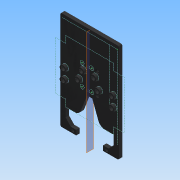
# Autodesk Inventor part: fix3
Saved by Autodesk Inventor 2015 (Build 190159000, 159)
## iProperties
Created: 2015-06-10
Part Number: fix3
Material: Générique
Document SubType Name: Modeling
Designer: Gregwar
Density: 1 g/cm^3
Appearance: Par défaut
Author: Gregwar
Autodesk Inventor part; units mm, degrees
ref_plane "YZ Plane" through (0, 0, 0) normal (1, 0, 0) x (0, 1, 0)
ref_plane "XZ Plane" through (0, 0, 0) normal (0, 1, 0) x (-1, 0, 0)
ref_plane "XY Plane" through (0, 0, 0) normal (0, 0, 1) x (1, 0, 0)
sketch "Esquisse1" plane through (0, 0, 0) normal (0, 1, 0) x (-1, 0, 0)
  line L0 (0, 0) -> (80, 0) construction
  line L1 (80, 0) -> (80, -120) construction
  line L2 (80, -120) -> (0, -120) construction
  line L3 (0, -120) -> (0, 0) construction
  line L4 (40, -120) -> (40, 0) construction
  line L5 (77.0201, -120) -> (40, -28.372) construction
  line L6 (75, 0) -> (75, -120) construction
  circle A0 centre (75, -60) radius 2.5 construction
  circle A1 centre (75, -75) radius 2.5 construction
  circle A2 centre (54.3966, -64.0049) radius 2.5 construction
  circle A3 centre (48.7775, -50.0971) radius 2.5 construction
  circle A4 centre (75, -20) radius 2 construction
  circle A5 centre (75, -5) radius 2 construction
  circle A6 centre (75, -115) radius 2 construction
  circle A7 centre (69.3809, -101.0922) radius 2 construction
  line L7 (75, -115) -> (69.3809, -101.0922) construction
  line L8 (52.7921, -43.0825) -> (41.0169, -47.84) construction
  line L9 (82.7607, -117.2572) -> (70.9854, -122.0147) construction
  line L10 (70.9854, -122.0147) -> (41.0169, -47.84) construction
  line L11 (82.7607, -117.2572) -> (52.7921, -43.0825) construction
  line L12 (54.3966, -64.0049) -> (69.3809, -101.0922) construction
  line L13 (67.7764, -80.1698) -> (56.0012, -84.9273) construction
  line L14 (81.35, 0) -> (68.65, 0) construction
  line L15 (68.65, 0) -> (68.65, -80) construction
  line L16 (68.65, -80) -> (81.35, -80) construction
  line L17 (81.35, -80) -> (81.35, 0) construction
  line L18 (75, 0) -> (75, -80) construction
  line L19 (75, -20) -> (75, -60) construction
  line L20 (2.9799, -120) -> (40, -28.372) construction
  line L21 (5, 0) -> (5, -120) construction
  circle A8 centre (5, -60) radius 2.5 construction
  circle A9 centre (5, -75) radius 2.5 construction
  circle A10 centre (25.6034, -64.0049) radius 2.5 construction
  circle A11 centre (31.2225, -50.0971) radius 2.5 construction
  circle A12 centre (5, -20) radius 2 construction
  circle A13 centre (5, -5) radius 2 construction
  circle A14 centre (5, -115) radius 2 construction
  circle A15 centre (10.6191, -101.0922) radius 2 construction
  line L22 (5, -115) -> (10.6191, -101.0922) construction
  line L23 (27.2079, -43.0825) -> (38.9831, -47.84) construction
  line L24 (9.0146, -122.0147) -> (38.9831, -47.84) construction
  line L25 (-2.7607, -117.2572) -> (27.2079, -43.0825) construction
  line L26 (25.6034, -64.0049) -> (10.6191, -101.0922) construction
  line L27 (12.2236, -80.1698) -> (23.9988, -84.9273) construction
  line L28 (11.35, 0) -> (11.35, -80) construction
  line L29 (11.35, -80) -> (-1.35, -80) construction
  line L30 (5, 0) -> (5, -80) construction
  line L31 (5, -20) -> (5, -60) construction
  point P0 (46.9045, -45.4612)
  point P1 (76.873, -119.6359)
  point P2 (61.8888, -82.5486)
  point P3 (75, -40)
  point P4 (33.0955, -45.4612)
  point P5 (18.1112, -82.5486)
  point P6 (5, -40)
  dimension "d0" = 80
  dimension "d1" = 120
  dimension "d2" = 5
  dimension "d3" = 4
  dimension "d4" = 15
  dimension "d5" = 15
  dimension "d6" = 40
  dimension "d7" = 5
  dimension "d8" = 5
  dimension "d9" = 15
  dimension "d10" = 40
  dimension "d11" = 15
  dimension "d12" = 5
  dimension "d13" = 5
  dimension "d14" = 68
  dimension "d15" = 12.7
  dimension "d17" = 80
  dimension "d18" = 12.7
  dimension "d19" = 80
  constraints: 64 end point, 25 symmetric about line, 21 point on line, 16 centre point, 14 midpoint, 7 parallel, 6 equal radius, 5 perpendicular, 2 horizontal, 1 collinear, 8 other
  measures "d0" distance of L0.start L0.end
  measures "d1" distance of L2.end L0.start
  measures "d2" diameter of A1
  measures "d3" diameter of A5
  measures "d4" distance of A1.centre L19.end
  measures "d5" distance of A5.centre L19.start
  measures "d6" distance of L19.start L19.end
  measures "d7" distance from line of L1 A5.centre
  measures "d8" distance from line of L0 A5.centre
  measures "d9" distance of L7.end L7.start
  measures "d10" distance of L12.start L7.end
  measures "d11" distance of A3.centre L12.start
  measures "d12" distance from line of L2 L7.start
  measures "d13" distance from line of L1 L7.start
  measures "d14" angle of L2 L5
  measures "d15" distance of L8.start L8.end
  measures "d17" distance of L9.start L8.start
  measures "d18" distance of L14.start L14.end
  measures "d19" distance of L14.end L15.end
sketch "Esquisse5" plane through (0, 0, 0) normal (0, 1, 0) x (-1, 0, 0)
  line L0 (5, -20) -> (75, -20)
  line L1 (75, -110) -> (5, -110)
  line L2 (90, -100) -> (90, -30)
  line L3 (-10, -30) -> (-10, -100)
  line L4 (75, -20) -> (75, -30)
  line L5 (75, -100) -> (75, -110)
  line L6 (90, -30) -> (75, -30)
  line L7 (5, -30) -> (-10, -30)
  line L8 (5, -110) -> (5, -100)
  line L9 (5, -30) -> (5, -20)
  line L10 (-10, -100) -> (5, -100)
  line L11 (75, -100) -> (90, -100)
  line L12 (40, -20) -> (40, -110) construction
  line L13 (40, -120) -> (40, 0) construction
  line L14 (0, 0) -> (80, 0) construction
  circle A0 centre (75, -60) radius 2.5 construction
  circle A1 centre (75, -75) radius 2.5 construction
  circle A2 centre (54.3966, -64.0049) radius 2.5 construction
  circle A3 centre (48.7775, -50.0971) radius 2.5 construction
  circle A4 centre (31.2225, -50.0971) radius 2.5 construction
  circle A5 centre (25.6034, -64.0049) radius 2.5 construction
  circle A6 centre (5, -60) radius 2.5 construction
  circle A7 centre (5, -75) radius 2.5 construction
  circle A8 centre (5, -60) radius 2.75
  circle A9 centre (5, -75) radius 2.75
  circle A10 centre (25.6034, -64.0049) radius 2.75
  circle A11 centre (31.2225, -50.0971) radius 2.75
  circle A12 centre (48.7775, -50.0971) radius 2.75
  circle A13 centre (54.3966, -64.0049) radius 2.75
  circle A14 centre (75, -60) radius 2.75
  circle A15 centre (75, -75) radius 2.75
  dimension "d37" = 100
  dimension "d38" = 90
  dimension "d39" = 10
  dimension "d40" = 15
  dimension "d41" = 20
  dimension "d42" = 5.5
  constraints: 26 end point, 10 parallel, 8 centre point, 8 coincident, 7 collinear, 7 equal radius, 4 perpendicular, 3 horizontal, 2 midpoint
  measures "d37" distance between parallel lines of L3 L2
  measures "d38" distance between parallel lines of L1 L0
  measures "d39" distance of L7.start L0.start
  measures "d40" distance of L2.end L4.end
  measures "d41" distance between parallel lines of L0 L14
  measures "d42" diameter of A9
extrude "Extrusion4" add sketch "Esquisse5" along normal blind 5
sketch "Esquisse6" plane through (0, 0, 0) normal (0, -1, 0) x (1, 0, 0)
  circle A0 centre (-75, -75) radius 2.75 construction
  circle A1 centre (-75, -60) radius 2.75 construction
  circle A2 centre (-54.3966, -64.0049) radius 2.75 construction
  circle A3 centre (-48.7775, -50.0971) radius 2.75 construction
  circle A4 centre (-31.2225, -50.0971) radius 2.75 construction
  circle A5 centre (-25.6034, -64.0049) radius 2.75 construction
  circle A6 centre (-5, -75) radius 2.75 construction
  circle A7 centre (-5, -60) radius 2.75 construction
  line L0 (-5, -20) -> (-75, -20) construction
  line L1 (-75, -20) -> (-75, -30) construction
  line L2 (-75, -30) -> (-90, -30) construction
  line L3 (-90, -30) -> (-90, -100) construction
  line L4 (-90, -100) -> (-75, -100) construction
  line L5 (-75, -100) -> (-75, -110) construction
  line L6 (-75, -110) -> (-5, -110) construction
  line L7 (-5, -110) -> (-5, -100) construction
  line L8 (-5, -100) -> (10, -100) construction
  line L9 (10, -100) -> (10, -30) construction
  line L10 (10, -30) -> (-5, -30) construction
  line L11 (-5, -30) -> (-5, -20) construction
  line L12 (-51, -42.5) -> (-37, -42.5) construction
  line L13 (-37, -42.5) -> (-37, -72.5) construction
  line L14 (-37, -72.5) -> (-51, -72.5) construction
  line L15 (-51, -72.5) -> (-51, -42.5) construction
  circle A8 centre (-51, -42.5) radius 1.2
  circle A9 centre (-37, -42.5) radius 1.2
  circle A10 centre (-37, -72.5) radius 1.2
  circle A11 centre (-51, -72.5) radius 1.2
  line L16 (-44, -42.5) -> (-44, -72.5) construction
  line L17 (-75, -20) -> (-5, -20) construction
  line L18 (-44, -20) -> (-44, -110) construction
  line L19 (-75, -110) -> (-5, -110) construction
  line L20 (-40, -20) -> (-40, -110) construction
  point P0 (0, 0)
  dimension "d45" = 14
  dimension "d46" = 30
  dimension "d47" = 2.4
  dimension "d48" = 22.5
  dimension "d127" = 4
  constraints: 14 end point, 4 centre point, 4 coincident, 4 midpoint, 3 equal radius, 2 parallel, 2 perpendicular, 2 point on line, 1 collinear, 1 horizontal
  measures "d45" distance of L12.start L12.end
  measures "d46" distance of L14.end L12.start
  measures "d47" diameter of A8
  measures "d48" distance between parallel lines of L0 L12
  measures "d127" distance between parallel lines of L18 L20
extrude "Extrusion5" cut sketch "Esquisse6" against normal through all
sketch "Esquisse7" plane through (0, 0, 0) normal (0, -1, 0) x (1, 0, 0)
  line L0 (-11.35, 0) -> (-11.35, -80) construction
  circle A0 centre (-37, -72.5) radius 1.2 construction
  circle A1 centre (-51, -42.5) radius 1.2 construction
  circle A2 centre (-37, -42.5) radius 1.2 construction
  circle A3 centre (-51, -72.5) radius 1.2 construction
  circle A4 centre (-75, -75) radius 2.75 construction
  circle A5 centre (-75, -60) radius 2.75 construction
  circle A6 centre (-54.3966, -64.0049) radius 2.75 construction
  circle A7 centre (-48.7775, -50.0971) radius 2.75 construction
  circle A8 centre (-31.2225, -50.0971) radius 2.75 construction
  circle A9 centre (-25.6034, -64.0049) radius 2.75 construction
  circle A10 centre (-5, -75) radius 2.75 construction
  circle A11 centre (-5, -60) radius 2.75 construction
  line L1 (-5, -20) -> (-75, -20) construction
  line L2 (-75, -20) -> (-75, -30) construction
  line L3 (-75, -30) -> (-90, -30) construction
  line L4 (-90, -30) -> (-90, -100) construction
  line L5 (-90, -100) -> (-75, -100) construction
  line L6 (-75, -100) -> (-75, -110) construction
  line L7 (-75, -110) -> (-5, -110) construction
  line L8 (-5, -110) -> (-5, -100) construction
  line L9 (-5, -100) -> (10, -100) construction
  line L10 (10, -100) -> (10, -30) construction
  line L11 (10, -30) -> (-5, -30) construction
  line L12 (-5, -30) -> (-5, -20) construction
  circle A12 centre (-51, -42.5) radius 1.2 projected
  circle A13 centre (-51, -42.5) radius 2
  circle A14 centre (-37, -42.5) radius 2
  circle A15 centre (-37, -72.5) radius 2
  circle A16 centre (-51, -72.5) radius 1.2 projected
  circle A17 centre (-51, -72.5) radius 2
  point P0 (0, 0)
  dimension "d51" = 4
  constraints: 4 centre point, 4 coincident, 3 equal radius
  measures "d51" diameter of A14
extrude "Extrusion6" cut sketch "Esquisse7" against normal blind 1
chamfer "Chanfrein1" distance 1 angle 45 4 edges at (-53, 0, -72.5) (-39, 0, -72.5) (-53, 0, -42.5) (-39, 0, -42.5)
sketch "Esquisse8" plane through (0, 0, 0) normal (0, -1, 0) x (1, 0, 0)
  circle A0 centre (-75, -60) radius 2.75 projected
  circle A1 centre (-75, -75) radius 2.75 projected
  circle A2 centre (-54.3966, -64.0049) radius 2.75 projected
  circle A3 centre (-48.7775, -50.0971) radius 2.75 projected
  circle A4 centre (-75, -60) radius 4.5
  circle A5 centre (-75, -75) radius 4.5
  circle A6 centre (-54.3966, -64.0049) radius 4.5
  circle A7 centre (-48.7775, -50.0971) radius 4.5
  line L0 (-40, -120) -> (-40, 0) construction
  circle A8 centre (-5, -60) radius 2.75
  circle A9 centre (-5, -75) radius 2.75
  circle A10 centre (-25.6034, -64.0049) radius 2.75
  circle A11 centre (-31.2225, -50.0971) radius 2.75
  circle A12 centre (-5, -60) radius 4.5
  circle A13 centre (-5, -75) radius 4.5
  circle A14 centre (-25.6034, -64.0049) radius 4.5
  circle A15 centre (-31.2225, -50.0971) radius 4.5
  point P0 (0, 0)
  dimension "d57" = 9
  constraints: 12 centre point, 8 coincident, 8 symmetric about line, 3 equal radius, 8 other
  measures "d57" diameter of A4
extrude "Extrusion7" add sketch "Esquisse8" along normal blind 4
sketch "Esquisse13" plane through (0, 0, 0) normal (0, -1, 0) x (1, 0, 0)
  circle A0 centre (-37, -72.5) radius 1.2 projected
  circle A1 centre (-51, -72.5) radius 1.2 projected
  circle A2 centre (-51, -72.5) radius 4.5
  circle A3 centre (-37, -72.5) radius 1.2 projected
  circle A4 centre (-37, -72.5) radius 4.5
  point P0 (0, 0)
  dimension "d77" = 9
  constraints: 2 centre point, 2 coincident, 1 equal radius
  measures "d77" diameter of A4
extrude "Extrusion10" cut sketch "Esquisse13" along normal through all contours A0 | A1 | A2 | A4
sketch "Esquisse15" plane through (0, 0, 0) normal (0, -1, 0) x (1, 0, 0)
  circle A0 centre (-51, -72.5) radius 3 construction
  circle A1 centre (-37, -72.5) radius 3 construction
  circle A2 centre (-25.6034, -64.0049) radius 4.5 construction
  circle A3 centre (-5, -60) radius 4.5 construction
  circle A4 centre (-54.3966, -64.0049) radius 4.5 construction
  circle A5 centre (-75, -60) radius 4.5 construction
  circle A6 centre (-75, -75) radius 4.5 construction
  circle A7 centre (-48.7775, -50.0971) radius 4.5 construction
  circle A8 centre (-5, -75) radius 4.5 construction
  circle A9 centre (-31.2225, -50.0971) radius 4.5 construction
  circle A10 centre (-51, -42.5) radius 3 construction
  line L0 (-5, -20) -> (-75, -20) construction
  line L1 (-75, -20) -> (-75, -30) construction
  line L2 (-75, -30) -> (-90, -30) construction
  line L3 (-90, -30) -> (-90, -100) construction
  line L4 (-90, -100) -> (-75, -100) construction
  line L5 (-75, -100) -> (-75, -110) construction
  line L6 (-75, -110) -> (-5, -110) construction
  line L7 (-5, -110) -> (-5, -100) construction
  line L8 (-5, -100) -> (10, -100) construction
  line L9 (10, -100) -> (10, -30) construction
  line L10 (10, -30) -> (-5, -30) construction
  line L11 (-5, -30) -> (-5, -20) construction
  circle A11 centre (-37, -42.5) radius 3 construction
  line L12 (-11.35, 0) -> (-11.35, -80) construction
  line L13 (0, -120) -> (0, 0) construction
  line L14 (0, 0) -> (-80, 0) construction
sketch "Esquisse17" plane through (0, 0, 0) normal (0, -1, 0) x (1, 0, 0)
  circle A0 centre (-37, -42.5) radius 3 construction
  circle A1 centre (-51, -42.5) radius 3 construction
  circle A2 centre (-31.2225, -50.0971) radius 4.5 construction
  circle A3 centre (-5, -75) radius 4.5 construction
  circle A4 centre (-48.7775, -50.0971) radius 4.5 construction
  circle A5 centre (-75, -75) radius 4.5 construction
  circle A6 centre (-75, -60) radius 4.5 construction
  circle A7 centre (-54.3966, -64.0049) radius 4.5 construction
  circle A8 centre (-5, -60) radius 4.5 construction
  circle A9 centre (-25.6034, -64.0049) radius 4.5 construction
  circle A10 centre (-37, -72.5) radius 3 construction
  circle A11 centre (-51, -72.5) radius 3 construction
  line L0 (-75, -110) -> (-5, -110) construction
  line L1 (-5, -110) -> (-5, -100) construction
  line L2 (-5, -100) -> (10, -100) construction
  line L3 (10, -100) -> (10, -30) construction
  line L4 (10, -30) -> (-5, -30) construction
  line L5 (-5, -30) -> (-5, -20) construction
  line L6 (-5, -20) -> (-75, -20) construction
  line L7 (-75, -20) -> (-75, -30) construction
  line L8 (-75, -30) -> (-90, -30) construction
  line L9 (-90, -30) -> (-90, -100) construction
  line L10 (-90, -100) -> (-75, -100) construction
  line L11 (-75, -100) -> (-75, -110) construction
  line L12 (-24.8691, -110) -> (-36.1818, -80)
  line L13 (-36.1818, -80) -> (-43.8182, -80)
  line L14 (-43.8182, -80) -> (-55.1309, -110)
  line L15 (-24.8691, -110) -> (-55.1309, -110)
  line L16 (-5, -110) -> (-75, -110) construction
  line L17 (-75, -100) -> (-90, -100) construction
  line L18 (-75, -20) -> (-5, -20)
  line L19 (-5, -20) -> (-5, -30)
  line L20 (-5, -30) -> (-75, -30)
  line L21 (-75, -30) -> (-75, -20)
  line L22 (-90, -100) -> (-75, -100) projected
  line L23 (-90, -30) -> (-82.5, -30)
  line L24 (-82.5, -30) -> (-82.5, -100)
  line L25 (-82.5, -100) -> (-90, -100)
  line L26 (-90, -100) -> (-90, -30)
  line L27 (-40, -20) -> (-40, -110) construction
  line L28 (10, -30) -> (10, -100) construction
  line L29 (10, -30) -> (2.5, -30)
  line L30 (2.5, -30) -> (2.5, -100)
  line L31 (2.5, -100) -> (10, -100)
  line L32 (10, -100) -> (10, -30)
  line L33 (-75, -110) -> (-5, -110) projected
  point P0 (0, 0)
  point P1 (-19.8008, -110)
  point P2 (-14.4081, -110)
  point P3 (-3.6724, -100)
  point P4 (-11.85, -20)
  point P5 (-15.85, -20)
  point P6 (-68.15, -20)
  point P7 (-76.3276, -100)
  point P8 (-65.5919, -110)
  point P9 (-60.1992, -110)
  dimension "d94" = 30
  constraints: 36 end point, 5 parallel, 4 symmetric about line, 3 horizontal, 3 midpoint, 2 perpendicular, 1 collinear
  measures "d94" distance between parallel lines of L15 L13
extrude "Extrusion12" cut sketch "Esquisse17" against normal through all
sketch "Esquisse18" plane through (0, 5, 0) normal (0, 1, 0) x (1, 0, 0)
  line L0 (2.5, 100) -> (-5, 100) construction
  line L1 (-5, 100) -> (-5, 110) construction
  line L2 (-5, 110) -> (-24.8691, 110) construction
  line L3 (-75, 110) -> (-75, 100) construction
  line L4 (-75, 100) -> (-82.5, 100) construction
  circle A0 centre (-37, 72.5) radius 1.2 construction
  circle A1 centre (-51, 42.5) radius 1.2 construction
  circle A2 centre (-37, 42.5) radius 1.2 construction
  circle A3 centre (-51, 72.5) radius 1.2 construction
  circle A4 centre (-75, 75) radius 2.75 construction
  circle A5 centre (-75, 60) radius 2.75 construction
  circle A6 centre (-54.3966, 64.0049) radius 2.75 construction
  circle A7 centre (-48.7775, 50.0971) radius 2.75 construction
  circle A8 centre (-31.2225, 50.0971) radius 2.75 construction
  circle A9 centre (-25.6034, 64.0049) radius 2.75 construction
  circle A10 centre (-5, 75) radius 2.75 construction
  circle A11 centre (-5, 60) radius 2.75 construction
  line L5 (-19.85, 30) -> (-60.15, 30) construction
  line L6 (-40, 30) -> (-40, 82) construction
  circle A12 centre (-75, 75) radius 5.05
  circle A13 centre (-75, 60) radius 5.05
  circle A14 centre (-54.3966, 64.0049) radius 2.75 projected
  circle A15 centre (-54.3966, 64.0049) radius 5.05
  circle A16 centre (-48.7775, 50.0971) radius 5.05
  line L7 (-44.5724, 82) -> (-35.4276, 82) construction
  line L8 (-35.4276, 82) -> (-24.1149, 110) construction
  line L9 (4.9558, 100) -> (1.7236, 92) construction
  line L10 (1.7236, 92) -> (1.7236, 42) construction
  line L11 (1.7236, 42) -> (5.5, 42) construction
  line L12 (5.5, 42) -> (5.5, 30) construction
  line L13 (5.5, 30) -> (-5, 30) construction
  line L14 (-5, 30) -> (-5, 20) construction
  line L15 (-19.85, 20) -> (-19.85, 30) construction
  line L16 (-19.85, 30) -> (-60.15, 30) construction
  circle A17 centre (-15.25, 95) radius 1.75 construction
  circle A18 centre (-29, 42.5) radius 1.2 construction
  circle A19 centre (-29, 72.5) radius 1.2 construction
  circle A20 centre (-5, 75) radius 2.75 construction
  circle A21 centre (-5, 60) radius 2.75 construction
  circle A22 centre (-25.6034, 64.0049) radius 2.75 construction
  circle A23 centre (-31.2225, 50.0971) radius 2.75 construction
  line L17 (-60.15, 30) -> (-19.85, 30) construction
  circle A24 centre (-5, 75) radius 5.05
  circle A25 centre (-5, 60) radius 5.05
  circle A26 centre (-25.6034, 64.0049) radius 2.75
  circle A27 centre (-25.6034, 64.0049) radius 5.05
  circle A28 centre (-31.2225, 50.0971) radius 5.05
  line L18 (-43.8182, 80) -> (-55.1309, 110) projected
  line L19 (-55.1309, 110) -> (-75, 110) projected
  line L20 (-24.8691, 110) -> (-36.1818, 80) projected
  line L21 (-36.1818, 80) -> (-43.8182, 80) projected
  line L22 (-82.5, 100) -> (-82.5, 30) projected
  line L23 (-82.5, 30) -> (2.5, 30) projected
  line L24 (2.5, 30) -> (2.5, 100) projected
  point P0 (0, 0)
  dimension "d104" = 10.1
  constraints: 24 end point, 16 centre point, 13 symmetric about line, 7 coincident, 3 equal radius, 1 midpoint, 11 other
  measures "d104" diameter of A12
extrude "Extrusion13" cut sketch "Esquisse18" against normal blind 2.7
chamfer "Chanfrein3" distance 1 angle 45 8 edges at (-10.05, 2.3, -75) (-10.05, 2.3, -60) (-30.6534, 2.3, -64.0049) (-36.2725, 2.3, -50.0971) (-53.8275, 2.3, -50.0971) (-59.4466, 2.3, -64.0049) (-80.05, 2.3, -75) (-80.05, 2.3, -60)
sketch "Esquisse20" plane through (0, 0, 0) normal (0, -1, 0) x (1, 0, 0)
  circle A0 centre (-37, -42.5) radius 3 construction
  circle A1 centre (-51, -42.5) radius 3 construction
  circle A2 centre (-31.2225, -50.0971) radius 4.5 construction
  circle A3 centre (-5, -75) radius 4.5 construction
  circle A4 centre (-48.7775, -50.0971) radius 4.5 construction
  circle A5 centre (-75, -75) radius 4.5 construction
  circle A6 centre (-75, -60) radius 4.5 construction
  circle A7 centre (-5, -60) radius 4.5 construction
  circle A8 centre (-25.6034, -64.0049) radius 4.5 construction
  circle A9 centre (-54.3966, -64.0049) radius 4.5 construction
  circle A10 centre (-37, -72.5) radius 3 construction
  circle A11 centre (-51, -72.5) radius 3 construction
  line L0 (-55.1309, -110) -> (-43.8182, -80) construction
  line L1 (-43.8182, -80) -> (-36.1818, -80) construction
  line L2 (-36.1818, -80) -> (-24.8691, -110) construction
  line L3 (-24.8691, -110) -> (-5, -110) construction
  line L4 (-5, -110) -> (-5, -100) construction
  line L5 (-5, -100) -> (2.5, -100) construction
  line L6 (2.5, -100) -> (2.5, -30) construction
  line L7 (2.5, -30) -> (-82.5, -30) construction
  line L8 (-82.5, -30) -> (-82.5, -100) construction
  line L9 (-82.5, -100) -> (-75, -100) construction
  line L10 (-75, -100) -> (-75, -110) construction
  line L11 (-75, -110) -> (-55.1309, -110) construction
  line L12 (-67.5, -92.5) -> (-12.5, -92.5) construction
  line L13 (-12.5, -92.5) -> (-12.5, -138) construction
  line L14 (-12.5, -138) -> (-67.5, -138) construction
  line L15 (-67.5, -138) -> (-67.5, -92.5) construction
  line L16 (-67.5, -135) -> (-12.5, -135) construction
  circle A12 centre (-64.5, -135) radius 1.7
  circle A13 centre (-15.5, -135) radius 1.7
  line L17 (-64.5, -135) -> (-15.5, -135) construction
  line L18 (-40, -80) -> (-40, -110) construction
  line L19 (-40, -92.5) -> (-40, -155.0345) construction
  line L20 (-67.5, -131) -> (-59.5, -131)
  line L21 (-59.5, -131) -> (-59.5, -138)
  line L22 (-82.5, -138) -> (-82.5, -100)
  line L23 (-82.5, -30) -> (-82.5, -100) projected
  line L24 (-67.5, -131) -> (-75, -123)
  line L25 (-75, -123) -> (-75, -110)
  line L26 (-75, -100) -> (-82.5, -100)
  line L27 (-59.5, -138) -> (-82.5, -138)
  line L28 (-75, -100) -> (-75, -110)
  line L29 (2.5, -100) -> (-5, -100) construction
  line L30 (-5, -100) -> (-5, -110) construction
  circle A14 centre (-15.5, -135) radius 1.7
  line L31 (-12.5, -131) -> (-20.5, -131)
  line L32 (-20.5, -131) -> (-20.5, -138)
  line L33 (2.5, -138) -> (2.5, -100)
  line L34 (-12.5, -131) -> (-5, -123)
  line L35 (-5, -123) -> (-5, -110)
  line L36 (-5, -100) -> (2.5, -100)
  line L37 (-20.5, -138) -> (2.5, -138)
  line L38 (-5, -100) -> (-5, -110)
  point P0 (0, 0)
  point P1 (-40, -135)
  dimension "d128" = 55
  dimension "d129" = 3
  dimension "d130" = 49
  dimension "d131" = 45.5
  dimension "d132" = 3.4
  dimension "d133" = 28
  dimension "d134" = 8
  dimension "d135" = 4
  dimension "d136" = 8
  constraints: 52 end point, 7 point on line, 5 symmetric about line, 4 collinear, 4 midpoint, 4 perpendicular, 3 centre point, 3 horizontal, 3 vertical, 2 parallel, 1 equal radius, 1 other
  measures "d128" distance of L13.end L14.end
  measures "d129" distance between parallel lines of L14 L16
  measures "d130" distance of L17.start L17.end
  measures "d131" distance of L14.end L12.start
  measures "d132" diameter of A12
  measures "d133" distance between parallel lines of L3 L14
  measures "d134" distance between parallel lines of L15 L21
  measures "d135" distance between parallel lines of L17 L20
  measures "d136" distance from line of L24.end L20
extrude "Extrusion15" add sketch "Esquisse20" against normal blind 5
fillet "Congé8" radius 10 2 edges at (-55.1309, 2.5, -110) (-24.8691, 2.5, -110)
sketch "Esquisse24" plane through (0, 5, 0) normal (0, 1, 0) x (1, 0, 0)
  arc A0 (-17.9526, 110) -> (-27.3095, 103.5284) centre (-17.9526, 100) ccw construction
  line L0 (-27.3095, 103.5284) -> (-36.1818, 80) construction
  line L1 (-36.1818, 80) -> (-43.8182, 80) construction
  line L2 (-43.8182, 80) -> (-52.6905, 103.5284) construction
  arc A1 (-52.6905, 103.5284) -> (-62.0474, 110) centre (-62.0474, 100) ccw construction
  line L3 (-62.0474, 110) -> (-75, 110) construction
  line L4 (-75, 110) -> (-75, 123) construction
  line L5 (-75, 123) -> (-67.5, 131) construction
  line L6 (-67.5, 131) -> (-59.5, 131) construction
  line L7 (-59.5, 131) -> (-59.5, 138) construction
  line L8 (-59.5, 138) -> (-82.5, 138) construction
  line L9 (-82.5, 138) -> (-82.5, 30) construction
  line L10 (-82.5, 30) -> (2.5, 30) construction
  line L11 (2.5, 30) -> (2.5, 138) construction
  line L12 (2.5, 138) -> (-20.5, 138) construction
  line L13 (-20.5, 138) -> (-20.5, 131) construction
  line L14 (-20.5, 131) -> (-12.5, 131) construction
  line L15 (-12.5, 131) -> (-5, 123) construction
  line L16 (-5, 123) -> (-5, 110) construction
  line L17 (-5, 110) -> (-17.9526, 110) construction
  circle A2 centre (-15.5, 135) radius 1.7 construction
  circle A3 centre (-64.5, 135) radius 1.7 construction
  circle A4 centre (-5, 60) radius 5.05 construction
  circle A5 centre (-25.6034, 64.0049) radius 5.05 construction
  circle A6 centre (-54.3966, 64.0049) radius 5.05 construction
  circle A7 centre (-75, 75) radius 5.05 construction
  circle A8 centre (-75, 60) radius 5.05 construction
  circle A9 centre (-48.7775, 50.0971) radius 5.05 construction
  circle A10 centre (-31.2225, 50.0971) radius 5.05 construction
  circle A11 centre (-5, 75) radius 5.05 construction
  circle A12 centre (-37, 72.5) radius 1.2 construction
  circle A13 centre (-51, 42.5) radius 1.2 construction
  circle A14 centre (-37, 42.5) radius 1.2 construction
  circle A15 centre (-51, 72.5) radius 1.2 construction
  line L18 (2.5, 30) -> (-82.5, 30)
  line L19 (-82.5, 30) -> (-82.5, -5)
  line L20 (-82.5, -5) -> (2.5, -5)
  line L21 (2.5, -5) -> (2.5, 30)
  line L22 (-82.5, 138) -> (-82.5, 30) projected
  point P0 (0, 0)
  dimension "d153" = 35
  constraints: 8 end point, 2 parallel, 1 collinear, 1 horizontal, 1 perpendicular
  measures "d153" distance between parallel lines of L10 L20
extrude "Extrusion18" add sketch "Esquisse24" against normal blind 5
fillet "Congé9" radius 2 4 edges at (2.5, 2.5, -138) (-82.5, 2.5, -138) (-82.5, 2.5, 5) (2.5, 2.5, 5)
ref_plane "Plan de construction1" through (-40, 0, -136) normal (-1, 0, 0) x (0, 0, 1)
mirror "Symétrie1" about plane through (-40, 0, -136) normal (-1, 0, 0) of "Extrusion5", "Extrusion6", "Chanfrein1"
equation "\"d5\" = d4"
equation "\"d8\" = d7"
equation "\"d12\" = d7"
equation "\"d13\" = d7"
